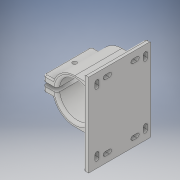
# Autodesk Inventor part: GeoPhoneSupport2
Saved by Autodesk Inventor 2019 (Build 230136000, 136)
## iProperties
Created: 2018-08-05
Part Number: GeoPhoneSupport2
Material: Generic
Document SubType Name: Modeling
Designer: Jia Ji
Density: 1 g/cm^3
Appearance: Default
Author: Jia Ji
Autodesk Inventor part; units mm, degrees
ref_plane "YZ Plane" through (0, 0, 0) normal (1, 0, 0) x (0, 1, 0)
ref_plane "XZ Plane" through (0, 0, 0) normal (0, 1, 0) x (-1, 0, 0)
ref_plane "XY Plane" through (0, 0, 0) normal (0, 0, 1) x (1, 0, 0)
sketch "Sketch1" plane through (0, 0, 0) normal (0, 0, 1) x (1, 0, 0)
  arc A0 (-12.913172, -1.5) -> (-12.913172, 1.5) centre (0, 0) ccw
  line L0 (16, 30) -> (20, 30)
  line L1 (20, 30) -> (20, -30)
  line L2 (20, -30) -> (16, -30)
  line L3 (16, -30) -> (16, 30)
  line L4 (0, 16) -> (16, 16)
  line L5 (0, -16) -> (16, -16)
  line L6 (-23, 5.5) -> (-15.024979, 5.5)
  line L7 (-12.913172, 1.5) -> (-23, 1.5)
  line L8 (-23, 1.5) -> (-23, 5.5)
  line L9 (-23, -1.5) -> (-12.913172, -1.5)
  line L10 (-15.024979, -5.5) -> (-23, -5.5)
  line L11 (-23, -5.5) -> (-23, -1.5)
  arc A1 (0, 16) -> (-15.024979, 5.5) centre (0, 0) ccw
  arc A2 (-15.024979, -5.5) -> (0, -16) centre (0, 0) ccw
  dimension "d0" = 26
  dimension "d2" = 4
  dimension "d3" = 60
  dimension "d4" = 30
  dimension "d5" = 16
  dimension "d6" = 4
  dimension "d7" = 4
  dimension "d8" = 1.5
  dimension "d9" = 1.5
  dimension "d64" = 23
  constraints: 24 end point, 6 point on circle, 4 horizontal, 4 parallel, 3 centre point, 2 perpendicular, 2 point on line, 2 tangent, 1 coincident, 1 collinear
  measures "d0" diameter of A0
  measures "d2" distance of L1.end L2.end
  measures "d3" distance of L0.end L1.end
  measures "d4" distance from line of point (0, 0) L0
  measures "d5" distance from line of L3 A0.centre
  measures "d6" distance between parallel lines of L7 L6
  measures "d7" distance between parallel lines of L10 L9
  measures "d8" distance from line of point (0, 0) L9
  measures "d9" distance from line of point (0, 0) L7
  measures "d64" distance from line of point (0, 0) L8
extrude "Extrusion1" add sketch "Sketch1" along normal blind 35 contours A0 L7 L8 L6 A1 L4 L3 L5 A2 L10 L11 L9
extrude "Extrusion2" add sketch "Sketch1" along normal blind 45 contours L3 L0 L1 L2
sketch "Sketch2" plane through (16, -30, 0) normal (-1, 0, 0) x (0, 0, 1)
  arc A0 (32.999245, 52.5) -> (32.999245, 55.5) centre (32.999245, 54) ccw
  arc A1 (29.999245, 55.5) -> (29.999245, 52.5) centre (29.999245, 54) ccw
  line L0 (32.999245, 55.5) -> (29.999245, 55.5)
  line L1 (32.999245, 52.5) -> (29.999245, 52.5)
  line L2 (44.999245, 0) -> (44.999245, 60)
  line L3 (44.999245, 60) -> (-0.000755, 60)
  arc A2 (12.999245, 52.5) -> (12.999245, 55.5) centre (12.999245, 54) ccw
  arc A3 (9.999245, 55.5) -> (9.999245, 52.5) centre (9.999245, 54) ccw
  line L4 (12.999245, 55.5) -> (9.999245, 55.5)
  line L5 (12.999245, 52.5) -> (9.999245, 52.5)
  arc A4 (32.999245, 4.5) -> (32.999245, 7.5) centre (32.999245, 6) ccw
  arc A5 (29.999245, 7.5) -> (29.999245, 4.5) centre (29.999245, 6) ccw
  line L6 (32.999245, 7.5) -> (29.999245, 7.5)
  line L7 (32.999245, 4.5) -> (29.999245, 4.5)
  line L8 (-0.000755, 0) -> (44.999245, 0)
  line L9 (-0.000755, 13.8) -> (-0.000755, 2)
  line L10 (-0.000755, 0) -> (-0.000755, 60)
  line L11 (12.999245, 7.5) -> (9.999245, 7.5)
  line L12 (12.999245, 4.5) -> (9.999245, 4.5)
  arc A6 (12.999245, 4.5) -> (12.999245, 7.5) centre (12.999245, 6) ccw
  arc A7 (9.999245, 7.5) -> (9.999245, 4.5) centre (9.999245, 6) ccw
  arc A8 (40.499245, 54) -> (37.499245, 54) centre (38.999245, 54) ccw
  line L13 (40.499245, 54) -> (40.499245, 51)
  line L14 (37.499245, 54) -> (37.499245, 51)
  arc A9 (37.499245, 51) -> (40.499245, 51) centre (38.999245, 51) ccw
  arc A10 (37.499245, 6) -> (40.499245, 6) centre (38.999245, 6) ccw
  line L15 (37.499245, 9) -> (37.499245, 6)
  line L16 (40.499245, 9) -> (40.499245, 6)
  arc A11 (40.499245, 9) -> (37.499245, 9) centre (38.999245, 9) ccw
  arc A12 (2.499245, 6) -> (5.499245, 6) centre (3.999245, 6) ccw
  line L17 (2.499245, 9) -> (2.499245, 6)
  line L18 (5.499245, 9) -> (5.499245, 6)
  arc A13 (5.499245, 9) -> (2.499245, 9) centre (3.999245, 9) ccw
  arc A14 (2.499245, 51) -> (5.499245, 51) centre (3.999245, 51) ccw
  line L19 (2.499245, 54) -> (2.499245, 51)
  line L20 (5.499245, 54) -> (5.499245, 51)
  arc A15 (5.499245, 54) -> (2.499245, 54) centre (3.999245, 54) ccw
  line L21 (0, 0) -> (45, 0)
  point P0 (0, 30)
  point P1 (-0.000755, 30.001124)
  point P2 (28.499245, 6)
  point P3 (14.499245, 6)
  point P4 (8.499245, 6)
  dimension "d16" = 3
  dimension "d17" = 3
  dimension "d18" = 3
  dimension "d19" = 12
  dimension "d20" = 6
  dimension "d21" = 3
  dimension "d22" = 3
  dimension "d23" = 3
  dimension "d24" = 3
  dimension "d25" = 3
  dimension "d26" = 3
  dimension "d27" = 6
  dimension "d28" = 12
  dimension "d29" = 3
  dimension "d30" = 3
  dimension "d31" = 3
  dimension "d32" = 10
  dimension "d33" = 10
  dimension "d34" = 6
  dimension "d35" = 6
  dimension "d36" = 6
  dimension "d37" = 3
  dimension "d38" = 3
  dimension "d39" = 3
  dimension "d40" = 6
  dimension "d41" = 3
  dimension "d42" = 3
  dimension "d43" = 3
  dimension "d44" = 3
  dimension "d45" = 3
  dimension "d46" = 3
  dimension "d47" = 3
  dimension "d48" = 3
  dimension "d49" = 3
  dimension "d50" = 6
  dimension "d51" = 4
  dimension "d52" = 4
  dimension "d53" = 6
  dimension "d54" = 6
  dimension "d55" = 6
  dimension "d58" = 60
  dimension "d59" = 45
  dimension "d60" = 60
  dimension "d61" = 6
  constraints: 42 end point, 35 point on circle, 16 centre point, 16 tangent, 4 perpendicular
  measures "d16" diameter of A0
  measures "d17" diameter of A1
  measures "d18" distance of A1.centre A0.centre
  measures "d19" distance from line of L2 A0.centre
  measures "d20" distance from line of A0.centre L3
  measures "d21" diameter of A2
  measures "d22" diameter of A3
  measures "d23" distance of A3.centre A2.centre
  measures "d24" diameter of A4
  measures "d25" diameter of A5
  measures "d26" distance of A5.centre A4.centre
  measures "d27" distance from line of L8 A4.centre
  measures "d28" distance from line of L2 A4.centre
  measures "d29" diameter of A6
  measures "d30" diameter of A7
  measures "d31" distance of A7.centre A6.centre
  measures "d32" distance from line of L10 A7.centre
  measures "d33" distance from line of L10 A3.centre
  measures "d34" distance from line of L3 A3.centre
  measures "d35" distance from line of L3 A2.centre
  measures "d36" distance from line of L8 A6.centre
  measures "d37" diameter of A8
  measures "d38" diameter of A9
  measures "d39" distance of A9.centre A8.centre
  measures "d40" distance from line of L2 A8.centre
  measures "d41" diameter of A11
  measures "d42" diameter of A10
  measures "d43" distance of A10.centre A11.centre
  measures "d44" diameter of A13
  measures "d45" diameter of A12
  measures "d46" distance of A12.centre A13.centre
  measures "d47" diameter of A15
  measures "d48" diameter of A14
  measures "d49" distance of A14.centre A15.centre
  measures "d50" distance from line of L3 A15.centre
  measures "d51" distance from line of L10 A15.centre
  measures "d52" distance from line of L9 A12.centre
  measures "d53" distance from line of L8 A12.centre
  measures "d54" distance from line of L8 A10.centre
  measures "d55" distance from line of L2 A10.centre
  measures "d58" distance between parallel lines of L21 L3
  measures "d59" distance between parallel lines of L10 L2
  measures "d60" distance between parallel lines of L8 L3
  measures "d61" distance from line of L8 A7.centre
extrude "Extrusion3" cut sketch "Sketch2" against normal blind 5 contours L1 A1 L0 A0 | L5 A3 L4 A2 | L7 A5 L6 A4 | A6 L12 A7 L11 | L13 A9 L14 A8 | L15 A11 L16 A10 | L17 A13 L18 A12 | L19 A15 L20 A14
sketch "Sketch4" plane through (-23, -5.5, 0) normal (0, -1, 0) x (1, 0, 0)
  circle A0 centre (4.4, 16.5) radius 2
  circle A1 centre (4.4, 16.5) radius 1.5
  line L0 (23, 0) -> (23, 35) projected
  dimension "d65" = 4
  dimension "d66" = 3
  dimension "d73" = 18.6
  constraints: 2 centre point, 1 coincident
  measures "d65" diameter of A0
  measures "d66" diameter of A1
  measures "d73" distance from line of L0 A0.centre
extrude "Extrusion4" cut sketch "Sketch4" against normal blind 15 contours A1
extrude "Extrusion5" cut sketch "Sketch4" against normal blind 5
fillet "Fillet1" radius 2 8 edges at (16, 0, 45) (16, -30, 22.5) (16, 30, 22.5) (13, 0, 35) (-23, 3.5, 35) (-23, -3.5, 35) (-23, -3.5, 0) (-23, 3.5, 0)
fillet "Fillet4" radius 1 2 edges at (16, -16, 17.5) (16, 16, 17.5)
sketch "Sketch7" plane through (-21, 1.5, 0) normal (0, -1, 0) x (1, 0, 0)
  line L0 (8.086828, 0) -> (34, 0)
  line L1 (8.086828, 0) -> (9.086828, 0)
  line L2 (9.086828, 0) -> (9.086828, 1)
  line L3 (9.086828, 1) -> (8.086828, 1)
  line L4 (8.086828, 1) -> (8.086828, 0)
  point P0 (21, 0)
  dimension "d79" = 1
  dimension "d80" = 1
  constraints: 8 end point, 2 parallel, 1 horizontal, 1 perpendicular
  measures "d79" distance of L3.end L2.end
  measures "d80" distance of L2.end L1.end
sketch "Sketch8" plane through (0, 0, 0) normal (0, 0, -1) x (-1, 0, 0)
  arc A0 (12.913172, 1.5) -> (12.913172, -1.5) centre (0, 0) ccw
  arc A1 (12.913172, 1.5) -> (12.913172, -1.5) centre (0, 0) ccw
  line L0 (12.913172, -1.5) -> (21, -1.5)
  line L1 (21, 1.5) -> (12.913172, 1.5)
  constraints: 2 end point, 2 point on circle, 1 centre point, 1 coincident
sketch3d "3D Sketch1"
  arc A0 (-12.913172, 1.5, 0) -> (0.751255, 12.978275, 0) centre (0, 0, 0) ccw
  arc A1 (0.751255, 12.978275, 0) -> (13, 0, 0) centre (0, 0, 0) ccw
  arc A2 (13, 0, 0) -> (0.751255, -12.978275, 0) centre (0, 0, 0) ccw
  arc A3 (0.751255, -12.978275, 0) -> (-12.913172, -1.5, 0) centre (0, 0, 0) ccw
sweep "Sweep1" add profiles "Sketch7" path "3D Sketch1"
fillet "Fillet5" radius 1 2 edges at (8.8111, 8.1571, 1) (-7.811, -9.1193, 1)
fillet "Fillet6" radius 1 22 edges at (15.7071, -16.2929, 0) (16, 22.5, 0) (16, -22.5, 0) (16.5858, -29.4142, 0) (19, -30, 0) (-9.1652, -13.1149, 0) (7.5, -16, 0) (-9.1652, 13.1149, 0) (15.7071, 16.2929, 0) (16.5858, 29.4142, 0) (19, 30, 0) (7.5, 16, 0) (-22.4142, -5.5, 34.4142) (-18.0125, -5.5, 35) (-22.4142, -5.5, 0.5858) (-18.0125, -5.5, 0) (-23, -5.5, 17.5) (-22.4142, 5.5, 34.4142) (-18.0125, 5.5, 35) (-22.4142, 5.5, 0.5858) (-18.0125, 5.5, 0) (-23, 5.5, 17.5)
body "Solid1"
